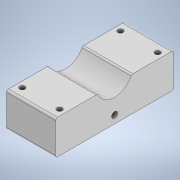
# Autodesk Inventor part: LowerSupport
Saved by Autodesk Inventor 2022 (Build 260153000, 153)
## iProperties
Created: 2021-11-02
Part Number: LowerSupport
Material: Genérico
Document SubType Name: Modeling
Designer: JK
Density: 1 g/cm^3
Appearance: Valor por defecto
Author: JK
Autodesk Inventor part; units mm, degrees
ref_plane "YZ Plane" through (0, 0, 0) normal (1, 0, 0) x (0, 1, 0)
ref_plane "XZ Plane" through (0, 0, 0) normal (0, 1, 0) x (-1, 0, 0)
ref_plane "XY Plane" through (0, 0, 0) normal (0, 0, 1) x (1, 0, 0)
sketch "Boceto1" plane through (0, 0, 0) normal (0, 1, 0) x (-1, 0, 0)
  line L0 (-25, 60) -> (25, 60)
  line L1 (25, 60) -> (25, -60)
  line L2 (25, -60) -> (-25, -60)
  line L3 (-25, -60) -> (-25, 60)
  line L4 (-25, 60) -> (25, -60) construction
  line L5 (25, 60) -> (-25, -60) construction
  circle A0 centre (19, 50) radius 2.7
  circle A1 centre (-19, 50) radius 2.7
  circle A2 centre (19, -50) radius 2.7
  circle A3 centre (-19, -50) radius 2.7
  point P0 (0, 0)
  dimension "d0" = 120
  dimension "d1" = 50
  dimension "d2" = 5.4
  dimension "d3" = 6
  dimension "d4" = 6
  dimension "d5" = 10
  dimension "d6" = 10
  dimension "d7" = 10
  constraints: 12 end point, 4 centre point, 3 equal radius, 2 midpoint, 2 parallel, 2 vertical alignment, 1 horizontal, 1 horizontal alignment, 1 perpendicular
  measures "d0" distance of L0.end L1.end
  measures "d1" distance between parallel lines of L3 L1
  measures "d2" diameter of A0
  measures "d3" distance from line of L1 A0.centre
  measures "d4" distance from line of L3 A1.centre
  measures "d5" distance from line of L0 A1.centre
  measures "d6" distance from line of L0 A0.centre
  measures "d7" distance from line of L2 A2.centre
extrude "Extrusión1" add sketch "Boceto1" along normal blind 35
sketch "Boceto2" plane through (-25, 0, -60) normal (-1, 0, 0) x (0, 0, 1)
  circle A0 centre (60, 8) radius 3
  line L0 (0, 0) -> (120, 0) projected
  line L1 (120, 0) -> (0, 0) projected
  point P0 (60, 0)
  point P1 (60, 0)
  dimension "d10" = 6
  dimension "d11" = 8
  constraints: 1 centre point, 1 midpoint, 1 vertical alignment
  measures "d10" diameter of A0
  measures "d11" distance from line of A0.centre L0
extrude "Extrusión2" cut sketch "Boceto2" against normal through all
sketch "Boceto3" plane through (25, 0, 60) normal (1, 0, 0) x (0, 0, -1)
  circle A0 centre (60, 42.6) radius 12.5
  line L0 (0, 35) -> (120, 35) projected
  line L1 (0, 0) -> (120, 0) projected
  point P0 (60, 0)
  point P1 (60, 0)
  dimension "d14" = 25
  dimension "d15" = 7.6
  constraints: 1 centre point, 1 midpoint, 1 vertical alignment
  measures "d14" diameter of A0
  measures "d15" distance from line of L0 A0.centre
extrude "Extrusión3" cut sketch "Boceto3" against normal through all
sketch "Boceto4" plane through (25, 0, 60) normal (1, 0, 0) x (0, 0, -1)
  circle A0 centre (60, 42.6) radius 18 projected
  point P0 (60, 0)
extrude "Extrusión4" cut sketch "Boceto4" against normal blind 104.5
sketch "Boceto5" plane through (25, 0, 60) normal (1, 0, 0) x (0, 0, -1)
  arc A0 (43.6831, 35) -> (76.3169, 35) centre (60, 42.6) ccw projected
  circle A1 centre (60, 42.6) radius 19
  point P0 (60, 0)
  dimension "d20" = 1
  constraints: 1 centre point, 1 coincident
  measures "d20" radial gap between concentric circles of A0 A1
extrude "Extrusión5" cut sketch "Boceto5" against normal through all
fillet "Empalme1" radius 2 6 edges at (0, 0, 60) (0, 35, 60) (0, 35, -60) (0, 0, -60) (0, 35, -17.4138) (0, 35, 17.4138)
